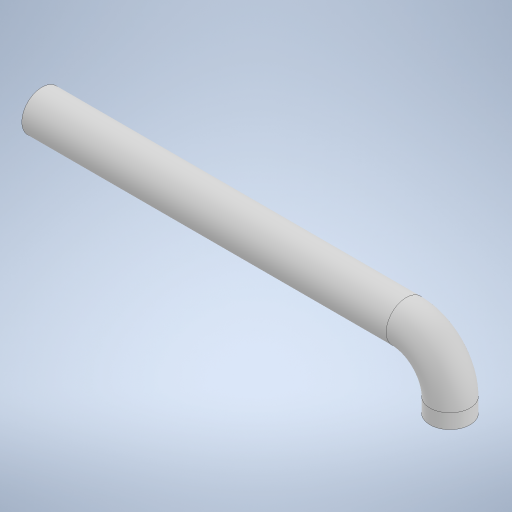
# Autodesk Inventor part: PenetrationUpstream
Saved by Autodesk Inventor 2023 (Build 270158000, 158)
## iProperties
Created: 2023-01-25
Part Number: PenetrationUpstream
Material: Generic
Document SubType Name: Modeling
Designer: remidm
Density: 1 g/cm^3
Appearance: Default
PenetrationUpstreamInnerDiameter: 0.197 in
PenetrationUpstreamThickness: 0.039 in
PenetrationUpstreamDistanceFromWallToCentre: 0.400 in
Author: remidm
Autodesk Inventor part; units mm, degrees
ref_plane "YZ Plane" through (0, 0, 0) normal (1, 0, 0) x (0, 1, 0)
ref_plane "XZ Plane" through (0, 0, 0) normal (0, 1, 0) x (-1, 0, 0)
ref_plane "XY Plane" through (0, 0, 0) normal (0, 0, 1) x (1, 0, 0)
sketch "Sketch1" plane through (0, 0, 0) normal (0, 1, 0) x (-1, 0, 0)
  circle A0 centre (0, 0) radius 2.5
  circle A1 centre (0, 0) radius 3.5
  dimension "PenetrationUpstreamInnerDiameter" = 5
  dimension "PenetrationUpstreamThickness" = 1
  constraints: 2 centre point, 2 coincident
  measures "PenetrationUpstreamInnerDiameter" diameter of A0
  measures "PenetrationUpstreamThickness" radial gap between concentric circles of A1 A0
sketch "Sketch2" plane through (0, 0, 0) normal (0, 0, 1) x (1, 0, 0)
  line L0 (-7.62, 10.16) -> (-71.12, 10.16)
  line L1 (0, 0) -> (0, 2.54)
  arc A0 (0, 2.54) -> (-7.62, 10.16) centre (-7.62, 2.54) ccw
  dimension "PenetrationUpstreamLength" = 63.5
  dimension "d14" = 90
  dimension "PenetrationUpstreamDistanceFromWallToCentre" = 10.16
  dimension "StraightBit" = 2.54
  constraints: 4 end point, 2 point on circle, 1 centre point, 1 coincident, 1 horizontal, 1 tangent, 1 vertical
  measures "PenetrationUpstreamLength" distance of L0.start L0.end
  measures "PenetrationUpstreamDistanceFromWallToCentre" distance from line of L1.start L0
  measures "StraightBit" distance of L1.start L1.end
sweep "Sweep2" add profiles "Sketch1" path "Sketch2"
equation "\"StraightBit\" = 0.25 * PenetrationUpstreamDistanceFromWallToCentre"
body "Solid3"
